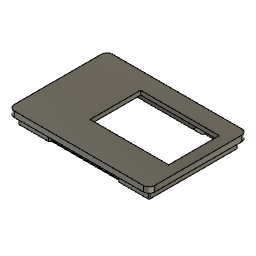
Air Unit Enclosure v9 (Autodesk Fusion 360 design; units mm, degrees)
Autodesk Fusion 360 part; units mm, degrees
sketch "Sketch2" plane through (0, 0, 0) normal (0, 0, 1) x (1, 0, 0) in component "Case"
  line L0 (0, 0) -> (50, 0)
  line L1 (50, 0) -> (50, 35)
  line L2 (50, 35) -> (0, 35)
  line L3 (0, 35) -> (0, 0)
  dimension "d14" = 50
  dimension "d15" = 35
  constraint horizontal L0
  constraint vertical L1
  constraint horizontal L2
  constraint vertical L3
  constraint coincident L0.start L3.end
  measures "d14" distance of L0.start L0.end
  measures "d15" distance of L0.start L2.end
extrude "Extrude3" add sketch "Sketch2" along normal blind 22 makes body 1 in component "Case"
fillet "Fillet2" radius 2 1 edges at (50, 0, 11) on bodies 1 in component "Case"
fillet "Fillet3" radius 2 1 edges at (0, 0, 11) on bodies 1 in component "Case"
fillet "Fillet4" radius 2 2 edges at (50, 35, 11) (0, 35, 11) on bodies 1 in component "Case"
shell "Shell2" thickness 1.5 removed faces 1 at (32.6667, 11.6667, 22) on bodies 1 in component "Case"
sketch "Sketch Nub protrusion" plane through (0, 1.5, 0) normal (0, 1, 0) x (-1, 0, 0) in component "Case"
  line L0 (-2, 1.5) -> (-2, 22)
  line L1 (-2, 22) -> (-48, 22)
  line L2 (-48, 22) -> (-48, 1.5)
  line L3 (-48, 1.5) -> (-2, 1.5)
  line L4 (-37.5, 22) -> (-12.5, 22)
  line L5 (-12.5, 22) -> (-12.5, 19)
  line L6 (-12.5, 19) -> (-37.5, 19)
  line L7 (-37.5, 19) -> (-37.5, 22)
  line L8 (-25, 22) -> (-25, 19) construction
  dimension "d22" = 25
  dimension "d23" = 3
  constraint horizontal L4
  constraint vertical L5
  constraint horizontal L6
  constraint vertical L7
  constraint coincident L1 L4.start
  constraint midpoint L1 L8.start
  constraint midpoint L6 L8.end
  constraint vertical L8
  measures "d22" distance of L4.start L4.end
  measures "d23" distance of L4.start L6.end
extrude "Extrude4" add sketch "Sketch Nub protrusion" along normal blind 6 draft -45 contours L1 L4 L5 L6 L7 bodies 1 in component "Case"
ref_plane "WorkPlane1" through (25, 17.5, 11) normal (0, -1, 0) x (1, 0, 0) in component "Case"
mirror "Mirror1" about plane through (25, 17.5, 11) normal (0, -1, 0) of "Extrude4" in component "Case"
sketch "Sketch1" plane through (0, 0, 22) normal (0, 0, 1) x (-1, 0, 0) in component "Top Cover"
  arc A0 (-1.5, -2) -> (-2, -1.5) centre (-2, -2) ccw
  line L0 (-1.5, -2) -> (-1.5, -33)
  arc A1 (-2, -33.5) -> (-1.5, -33) centre (-2, -33) ccw
  line L1 (-2, -33.5) -> (-12.5, -33.5)
  line L2 (-12.5, -33.5) -> (-37.5, -33.5)
  line L3 (-37.5, -33.5) -> (-48, -33.5)
  arc A2 (-48.5, -33) -> (-48, -33.5) centre (-48, -33) ccw
  line L4 (-48.5, -33) -> (-48.5, -2)
  arc A3 (-48, -1.5) -> (-48.5, -2) centre (-48, -2) ccw
  line L5 (-48, -1.5) -> (-37.5, -1.5)
  line L6 (-37.5, -1.5) -> (-12.5, -1.5)
  line L7 (-12.5, -1.5) -> (-2, -1.5)
  arc A4 (-2, -35) -> (0, -33) centre (-2, -33) ccw
  line L8 (0, -33) -> (0, -2)
  arc A5 (0, -2) -> (-2, 0) centre (-2, -2) ccw
  line L9 (-2, 0) -> (-48, 0)
  arc A6 (-48, 0) -> (-50, -2) centre (-48, -2) ccw
  line L10 (-50, -2) -> (-50, -33)
  arc A7 (-50, -33) -> (-48, -35) centre (-48, -33) ccw
  line L11 (-48, -35) -> (-2, -35)
extrude "Extrude1" add sketch "Sketch1" along normal blind 2 separate body contours A0 L0 A1 L1 L2 L3 A2 L4 A3 L5 L6 L7 | A4 L8 A5 L9 A6 L10 A7 L11 makes body 2 in component "Top Cover"
sketch "Sketch2 (2)" plane through (0, 0, 22) normal (0, 0, -1) x (1, 0, 0) in component "Top Cover"
  line L0 (2, -35) -> (48, -35)
  arc A0 (48, -35) -> (50, -33) centre (48, -33) ccw
  line L1 (50, -33) -> (50, -2)
  arc A1 (50, -2) -> (48, 0) centre (48, -2) ccw
  line L2 (48, 0) -> (2, 0)
  arc A2 (2, 0) -> (0, -2) centre (2, -2) ccw
  line L3 (0, -2) -> (0, -33)
  arc A3 (0, -33) -> (2, -35) centre (2, -33) ccw
  arc A4 (1.7, -33) -> (2, -33.3) centre (2, -33) ccw
  line L4 (2, -33.3) -> (48, -33.3)
  arc A5 (48, -33.3) -> (48.3, -33) centre (48, -33) ccw
  line L5 (48.3, -33) -> (48.3, -2)
  arc A6 (48.3, -2) -> (48, -1.7) centre (48, -2) ccw
  line L6 (48, -1.7) -> (2, -1.7)
  arc A7 (2, -1.7) -> (1.7, -2) centre (2, -2) ccw
  line L7 (1.7, -2) -> (1.7, -33)
extrude "Extrude4'" add sketch "Sketch2 (2)" along normal blind 3 contours A4 L4 A5 L5 A6 L6 A7 L7 bodies 2 in component "Top Cover"
extrude "Extrude2" add sketch "Sketch2 (2)" along normal blind 3 contours A4 L4 A5 L5 A6 L6 A7 L7 bodies 2 in component "Top Cover"
extrude "Extrude3'" cut sketch "Sketch Nub protrusion" along normal blind 3 draft -45 from surface at 0.2 contours L1 L4 L5 L6 L7 bodies 2 in component "Top Cover"
mirror "Mirror1'" about plane through (25, 17.5, 11) normal (0, -1, 0) of "Extrude3'" in component "Top Cover"
shell "Shell1" thickness 1.5 removed faces 1 at (29.1667, 22.7667, 19) on bodies 2 in component "Top Cover"
chamfer "Chamfer1" distance 0.6 angle 45 1 edges at (25, 33.3, 19) on bodies 2 in component "Top Cover"
chamfer "Chamfer2" distance 0.6 angle 45 1 edges at (25, 1.7, 19) on bodies 2 in component "Top Cover"
sketch "LCD Cutout" plane through (0, 0, 24) normal (0, 0, 1) x (-1, 0, 0) in component "Top Cover"
  line L0 (-48, -35) -> (-2, -35)
  arc A0 (-2, -35) -> (0, -33) centre (-2, -33) ccw
  line L1 (0, -33) -> (0, -2)
  arc A1 (0, -2) -> (-2, 0) centre (-2, -2) ccw
  line L2 (-2, 0) -> (-48, 0)
  arc A2 (-48, 0) -> (-50, -2) centre (-48, -2) ccw
  line L3 (-50, -2) -> (-50, -33)
  arc A3 (-50, -33) -> (-48, -35) centre (-48, -33) ccw
  line L4 (-18.1165, -28.8892) -> (-46.1165, -28.8892)
  line L5 (-46.1165, -28.8892) -> (-46.1165, -10.8892)
  line L6 (-46.1165, -10.8892) -> (-18.1165, -10.8892)
  line L7 (-18.1165, -10.8892) -> (-18.1165, -28.8892)
  dimension "d48" = 28
  dimension "d49" = 18
  constraint horizontal L4
  constraint vertical L5
  constraint horizontal L6
  constraint vertical L7
  measures "d48" distance of L4.start L4.end
  measures "d49" distance of L4.start L6.end
extrude "Extrude5" cut sketch "LCD Cutout" against normal blind 6 contours L4 L5 L6 L7 bodies 2 in component "Top Cover"
sketch "AntHole" plane through (0, 0, 0) normal (-1, 0, 0) x (0, -1, 0) in component "Case"
  line L0 (-33, 22) -> (-33, 0)
  line L1 (-33, 0) -> (-2, 0)
  line L2 (-2, 0) -> (-2, 22)
  line L3 (-2, 22) -> (-33, 22)
  line L4 (-17.5, 0) -> (-17.5, 22) construction
  line L5 (-33, 11) -> (-2, 11) construction
  circle A0 centre (-17.5, 11) radius 3 construction
  circle A1 centre (-17.5, 11) radius 3
  line L6 (-29, 13) -> (-26, 13)
  line L7 (-26, 13) -> (-26, 3)
  line L8 (-26, 3) -> (-29, 3)
  line L9 (-29, 3) -> (-29, 13)
  dimension "d52" = 6
  dimension "d55" = 3
  constraint midpoint L1 L4.start
  constraint midpoint L3 L4.end
  constraint midpoint L0 L5.start
  constraint midpoint L2 L5.end
  constraint midpoint L4 A0.centre
  constraint concentric A0 A1
  constraint horizontal L6
  constraint vertical L7
  constraint horizontal L8
  constraint vertical L9
  measures "d52" diameter of A0
  measures "d55" distance of L6.start L6.end
extrude "Extrude6" cut sketch "AntHole" against normal blind 3 contours L6 L7 L8 L9 bodies 1 in component "Case"
extrude "Extrude5'" cut sketch "AntHole" against normal blind 3 contours A1 bodies 1 in component "Case"
sketch "Sketch1 (2)" plane through (0, 0, 0) normal (0, 0, 1) x (1, 0, 0) in component "Case"
  line L0 (0, 0) -> (35, 0)
  line L1 (35, 0) -> (35, -50)
  line L2 (35, -50) -> (0, -50)
  line L3 (0, -50) -> (0, 0)
  dimension "d6" = 35
  dimension "d7" = 50
  constraint horizontal L0
  constraint vertical L1
  constraint horizontal L2
  constraint vertical L3
  constraint coincident L0.start L3.end
  measures "d6" distance of L0.start L0.end
  measures "d7" distance of L0.start L2.end
extrude "Extrude1'" [suppressed] in component "Case"
extrude "Extrude2'" [suppressed] in component "Case"
fillet "Fillet1" [suppressed] in component "Case"
shell "Shell1'" [suppressed] in component "Case"
component "Enclosure" placed x (1, 0, 0) y (0, 1, 0) z (0, 0, 1) at (0, 0, 0)
component "Case" placed x (1, 0, 0) y (0, 1, 0) z (0, 0, 1) at (0, 0, 0) in component "Enclosure"
component "Top Cover" placed x (1, 0, 0) y (0, 1, 0) z (0, 0, 1) at (0, 0, 0) in component "Enclosure"
equation "width = 35 mm"
equation "length = 50 mm"
equation "height = 22 mm"
equation "shell = 1.5 mm"
equation "gap = 0.2 mm"
equation "d6 = width"
equation "d7 = length"
equation "d8 = height"
equation "d10 = height"
equation "d13 = shell"
equation "d14 = length"
equation "d15 = width"
equation "d16 = height"
equation "d21 = shell"
equation "d22 = length / 2"
equation "d23 = shell * 2"
equation "d30 = -shell - gap"
equation "d31 = shell * 2"
equation "d34 = shell * 2"
equation "d36 = shell * 2"
equation "d40 = shell"
